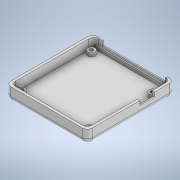
# Autodesk Inventor part: Enclosure Box
Saved by Autodesk Inventor 2021 (Build 250183000, 183)
## iProperties
Created: 2021-06-04
Part Number: Enclosure Box
Material: Generic
Document SubType Name: Modeling
Designer: Anton
Density: 1 g/cm^3
Appearance: Default
Author: Anton
Autodesk Inventor part; units mm, degrees
ref_plane "YZ Plane" through (0, 0, 0) normal (1, 0, 0) x (0, 1, 0)
ref_plane "XZ Plane" through (0, 0, 0) normal (0, 1, 0) x (-1, 0, 0)
ref_plane "XY Plane" through (0, 0, 0) normal (0, 0, 1) x (1, 0, 0)
sketch "Sketch2" plane through (0, 0, 0) normal (0, 1, 0) x (-1, 0, 0)
  line L0 (0, 0) -> (62, 0)
  line L1 (62, 0) -> (62, -66)
  line L2 (62, -66) -> (0, -66)
  line L3 (0, -66) -> (0, 0)
  circle A0 centre (58.15, -9.3) radius 1.5
  circle A1 centre (57.35, -60.86) radius 1.5
  circle A2 centre (3, -4.5) radius 1.5
  circle A3 centre (3, -61.9) radius 1.5
  circle A4 centre (3, -4.5) radius 3
  circle A5 centre (58.15, -9.3) radius 3
  circle A6 centre (57.35, -60.86) radius 3
  circle A7 centre (3, -61.9) radius 3
  line L4 (63, 20) -> (-1, 20)
  line L5 (-1, 20) -> (-1, -86)
  line L6 (-1, -86) -> (63, -86)
  line L7 (63, -86) -> (63, 20)
  dimension "d14" = 66
  dimension "d15" = 62
  dimension "d16" = 3
  dimension "d17" = 3
  dimension "d18" = 3
  dimension "d19" = 3
  dimension "d20" = 3
  dimension "d21" = 4.5
  dimension "d22" = 6
  dimension "d23" = 3
  dimension "d24" = 57.4
  dimension "d25" = 54.35
  dimension "d26" = 0.8
  dimension "d27" = 51.56
  dimension "d28" = 4.8
  dimension "d29" = 6
  dimension "d30" = 6
  dimension "d31" = 6
  dimension "d32" = 20
  dimension "d33" = 20
  dimension "d34" = 1
  dimension "d35" = 1
  constraints: 16 end point, 8 centre point, 4 coincident, 4 parallel, 2 horizontal, 2 perpendicular
  measures "d14" distance between parallel lines of L2 L0
  measures "d15" distance between parallel lines of L3 L1
  measures "d16" diameter of A0
  measures "d17" diameter of A1
  measures "d18" diameter of A3
  measures "d19" diameter of A2
  measures "d20" distance from line of L3 A2.centre
  measures "d21" distance from line of A2.centre L0
  measures "d22" diameter of A4
  measures "d23" distance from line of L3 A3.centre
  measures "d24" distance of A2.centre A3.centre
  measures "d25" horizontal distance of A1.centre A3.centre
  measures "d26" horizontal distance of A1.centre A0.centre
  measures "d27" vertical distance of A1.centre A0.centre
  measures "d28" vertical distance of A2.centre A0.centre
  measures "d29" diameter of A5
  measures "d30" diameter of A6
  measures "d31" diameter of A7
  measures "d32" distance between parallel lines of L4 L0
  measures "d33" distance between parallel lines of L2 L6
  measures "d34" distance between parallel lines of L7 L1
  measures "d35" distance between parallel lines of L3 L5
extrude "Extrusion1" add sketch "Sketch2" along normal blind 2 contours A4 | A7 | L0 L1 L2 L3 | A0 | A1 | A2 | A3 | A5 | A6
sketch "Sketch4" plane through (0, 2, 0) normal (0, 1, 0) x (1, 0, 0)
  line L0 (-62, 66) -> (0, 66)
  line L1 (0, 66) -> (0, 0)
  line L2 (0, 0) -> (-62, 0)
  line L3 (-62, 0) -> (-62, 66)
  circle A0 centre (-3.85, 56.7) radius 1.5
  circle A1 centre (-4.65, 5.14) radius 1.5
  circle A2 centre (-59, 61.5) radius 1.5
  circle A3 centre (-59, 4.1) radius 1.5
  circle A4 centre (-59, 61.5) radius 3
  circle A5 centre (-3.85, 56.7) radius 3
  circle A6 centre (-4.65, 5.14) radius 3
  circle A7 centre (-59, 4.1) radius 3
  point P0 (0, 0)
  dimension "d38" = 66
  dimension "d40" = 3
  dimension "d41" = 3
  dimension "d42" = 3
  dimension "d43" = 3
  dimension "d44" = 3
  dimension "d45" = 4.5
  dimension "d46" = 6
  dimension "d47" = 3
  dimension "d48" = 57.4
  dimension "d50" = 0.8
  dimension "d51" = 51.56
  dimension "d52" = 4.8
  dimension "d53" = 6
  dimension "d54" = 6
  dimension "d55" = 6
  constraints: 8 centre point, 8 end point, 4 coincident, 2 parallel, 1 horizontal, 1 perpendicular
  measures "d38" distance between parallel lines of L2 L0
  measures "d40" diameter of A0
  measures "d41" diameter of A1
  measures "d42" diameter of A3
  measures "d43" diameter of A2
  measures "d44" distance from line of L3 A2.centre
  measures "d45" distance from line of A2.centre L0
  measures "d46" diameter of A4
  measures "d47" distance from line of L3 A3.centre
  measures "d48" distance of A2.centre A3.centre
  measures "d50" horizontal distance of A1.centre A0.centre
  measures "d51" vertical distance of A1.centre A0.centre
  measures "d52" vertical distance of A2.centre A0.centre
  measures "d53" diameter of A5
  measures "d54" diameter of A6
  measures "d55" diameter of A7
extrude "Extrusion2" add sketch "Sketch4" along normal blind 3 contours A4 | A7 | A0 | A1 | A2 | A3 | A5 | A6
sketch "Sketch69" plane through (-59, 5, -4.1) normal (0, 1, 0) x (1, 0, 0)
  circle A0 centre (54.35, 1.04) radius 3 projected
  circle A1 centre (54.35, 1.04) radius 1.25
  circle A2 centre (55.15, 52.6) radius 3 projected
  circle A3 centre (55.15, 52.6) radius 1.25
  circle A4 centre (0, 57.4) radius 3 projected
  circle A5 centre (0, 57.4) radius 1.25
  circle A6 centre (0, 0) radius 3 projected
  circle A7 centre (0, 0) radius 1.25
  point P0 (59, -4.1)
  point P1 (-3, 57.4)
  point P2 (-3, 0)
  dimension "d432" = 2.5
  dimension "d433" = 2.5
  dimension "d434" = 2.5
  dimension "d435" = 2.5
  constraints: 4 centre point, 4 coincident, 2 horizontal alignment
  measures "d432" diameter of A7
  measures "d433" diameter of A5
  measures "d434" diameter of A3
  measures "d435" diameter of A1
extrude "Extrusion56" add sketch "Sketch69" along normal blind 3 contours A1 | A3 | A5 | A7
sketch "Sketch72" plane through (0, 2, 0) normal (0, 1, 0) x (1, 0, 0)
  line L0 (-62, 66) -> (-62, 0) projected
  line L1 (-62, 66) -> (-65, 66)
  line L2 (-65, 66) -> (-65, 0)
  line L3 (-65, 0) -> (-62, 0)
  line L4 (-62, 0) -> (-62, 66)
  circle A0 centre (-59, 61.5) radius 1.25 projected
  line L5 (0, 66) -> (-62, 66) projected
  line L6 (-62, 0) -> (0, 0) projected
  line L7 (0, 0) -> (2.15, 0)
  line L8 (2.15, 0) -> (2.15, 66)
  line L9 (2.15, 66) -> (0, 66)
  line L10 (0, 66) -> (0, 0)
  circle A1 centre (-3.85, 56.7) radius 1.25 projected
  line L11 (-65, 66) -> (2.15, 66)
  line L12 (2.15, 66) -> (2.15, 68.5)
  line L13 (2.15, 68.5) -> (-65, 68.5)
  line L14 (-65, 68.5) -> (-65, 66)
  line L15 (-65, 0) -> (2.15, 0)
  line L16 (2.15, 0) -> (2.15, -3)
  line L17 (2.15, -3) -> (-65, -3)
  line L18 (-65, -3) -> (-65, 0)
  circle A2 centre (-59, 4.1) radius 1.25 projected
  dimension "d446" = 6
  dimension "d447" = 0
  dimension "d448" = 6
  dimension "d449" = 7
  dimension "d450" = 7.1
  dimension "d464" = 0
  dimension "d465" = 0
  constraints: 32 end point, 8 parallel, 4 horizontal, 4 perpendicular, 1 point on line
  measures "d446" distance from line of A0.centre L2
  measures "d447" distance between parallel lines of L5 L1
  measures "d448" distance from line of L8 A1.centre
  measures "d449" distance from line of A0.centre L13
  measures "d450" distance from line of L17 A2.centre
  measures "d464" distance between parallel lines of L8 L12
  measures "d465" distance between parallel lines of L8 L16
extrude "Extrusion58" add sketch "Sketch72" against normal blind 2 contours L0 L3 L2 L1 | L1 L14 L13 L12 L9 L5 | L6 L7 L16 L17 L18 L3 | L9 L8 L7 L10
sketch "Sketch73" plane through (0, 2, 0) normal (0, 1, 0) x (1, 0, 0)
  line L0 (2.15, -3) -> (-65, -3) projected
  line L1 (-65, 68.5) -> (2.15, 68.5) projected
  line L2 (-65, -3) -> (2.15, -3)
  line L3 (2.15, -3) -> (2.15, 68.5)
  line L4 (2.15, 68.5) -> (-65, 68.5)
  line L5 (-65, 68.5) -> (-65, -3)
  line L6 (-63, -1) -> (0.15, -1)
  line L7 (0.15, -1) -> (0.15, 66.5)
  line L8 (0.15, 66.5) -> (-63, 66.5)
  line L9 (-63, 66.5) -> (-63, -1)
  point P0 (0, 0)
  point P1 (2.15, -3)
  dimension "d453" = 2
  constraints: 16 end point, 4 parallel, 2 perpendicular, 1 horizontal, 3 other
  measures "d453" distance between parallel lines of L5 L9
extrude "Extrusion59" add sketch "Sketch73" along normal blind 6
sketch "Sketch74" plane through (0, 8, 0) normal (0, 1, 0) x (1, 0, 0)
  line L0 (6.1553, 52.4) -> (-1.961, 52.4)
  line L1 (-1.961, 52.4) -> (-1.961, 40.4)
  line L2 (-1.961, 40.4) -> (6.1553, 40.4)
  line L3 (6.1553, 40.4) -> (6.1553, 52.4)
  line L4 (-3.5, 77.4858) -> (-56, 77.4858)
  line L5 (-56, 77.4858) -> (-56, 63.7045)
  line L6 (-56, 63.7045) -> (-3.5, 63.7045)
  line L7 (-3.5, 63.7045) -> (-3.5, 77.4858)
  circle A0 centre (-59, 61.5) radius 1.25 projected
  line L8 (0.15, -1) -> (0.15, 66.5) projected
  line L9 (-63, 67.5) -> (0.15, 67.5)
  line L10 (0.15, 67.5) -> (0.15, 64.6943)
  line L11 (0.15, 64.6943) -> (-63, 64.6943)
  line L12 (-63, 64.6943) -> (-63, 67.5)
  line L13 (-63, 66.5) -> (0.15, 66.5) projected
  circle A1 centre (-3.85, 56.7) radius 1.25 projected
  point P0 (0, 0)
  point P1 (-56, 64.6943)
  point P2 (-3.5, 64.6943)
  point P3 (-56, 66.5)
  point P4 (-56, 67.5)
  point P5 (-3.5, 66.5)
  point P6 (0.15, 66.5)
  point P7 (-3.5, 67.5)
  dimension "d457" = 52.5
  dimension "d458" = 1
  dimension "d459" = 4.3
  dimension "d460" = 12
  dimension "d463" = 3
  constraints: 24 end point, 6 parallel, 3 horizontal, 3 perpendicular, 1 point on line
  measures "d457" distance between parallel lines of L7 L5
  measures "d458" distance between parallel lines of L13 L9
  measures "d459" distance from line of L0 A1.centre
  measures "d460" distance between parallel lines of L0 L2
  measures "d463" distance from line of L5 A0.centre
extrude "Extrusion60" cut sketch "Sketch74" against normal blind 3 contours L3 L2 L8 L0 | L8 L2 L1 L0 | L7 L9 L5 L4 | L9 L10 L13 L7 | L7 L13 L5 L9 | L5 L13 L12 L9 | L7 L11 L5 L13
sketch "Sketch75" plane through (0, 5, 0) normal (0, 1, 0) x (1, 0, 0)
  line L0 (-56, 68.5) -> (-3.5, 68.5) projected
  line L1 (-56, 68.5) -> (-3.5, 68.5)
  line L2 (-3.5, 68.5) -> (-3.5, 67.5)
  line L3 (-3.5, 67.5) -> (-56, 67.5)
  line L4 (-56, 67.5) -> (-56, 68.5)
  point P0 (0, 0)
  point P1 (-3.5, 68.5)
  constraints: 8 end point, 2 parallel, 1 horizontal, 1 perpendicular
extrude "Extrusion61" add sketch "Sketch75" along normal blind 1.5
sketch "Sketch77" plane through (0, 5, 0) normal (0, 1, 0) x (1, 0, 0)
  line L0 (2.15, 52.4) -> (2.15, 68.5) projected
  line L1 (2.15, 40.4) -> (0.15, 40.4) projected
  line L2 (2.15, 52.4) -> (1.15, 52.4)
  line L3 (1.15, 52.4) -> (1.15, 40.4)
  line L4 (1.15, 40.4) -> (2.15, 40.4)
  line L5 (2.15, 40.4) -> (2.15, 52.4)
  point P0 (0, 0)
  dimension "d469" = 1
  constraints: 8 end point, 2 parallel, 1 horizontal, 1 midpoint, 1 perpendicular
  measures "d469" distance between parallel lines of L5 L3
extrude "Extrusion62" add sketch "Sketch77" along normal blind 1.5
sketch "Sketch78" plane through (0, 8, 0) normal (0, 1, 0) x (1, 0, 0)
  line L0 (2.15, 40.4) -> (0.15, 40.4) projected
  line L1 (0.15, 40.4) -> (0.15, -1) projected
  line L2 (0.15, -1) -> (-63, -1) projected
  line L3 (-63, -1) -> (-63, 67.5) projected
  line L4 (-63, 67.5) -> (-56, 67.5) projected
  line L5 (-56, 67.5) -> (-56, 68.5) projected
  line L6 (-56, 68.5) -> (-65, 68.5) projected
  line L7 (-65, 68.5) -> (-65, -3) projected
  line L8 (-65, -3) -> (2.15, -3) projected
  line L9 (2.15, -3) -> (2.15, 40.4) projected
  line L10 (0.15, 52.4) -> (2.15, 52.4) projected
  line L11 (2.15, 52.4) -> (2.15, 68.5) projected
  line L12 (2.15, 68.5) -> (-3.5, 68.5) projected
  line L13 (-3.5, 68.5) -> (-3.5, 67.5) projected
  line L14 (-3.5, 67.5) -> (0.15, 67.5) projected
  line L15 (0.15, 67.5) -> (0.15, 52.4) projected
  point P0 (0, 0)
extrude "Extrusion63" add sketch "Sketch78" along normal blind 2
sketch "Sketch80" plane through (0, 10, 0) normal (0, 1, 0) x (1, 0, 0)
  line L0 (2.15, -3) -> (-65, -3) projected
  line L1 (-1.85, -3) -> (-61, -3)
  line L2 (-65, 1) -> (-65, 64.5)
  line L3 (-61, 68.5) -> (-1.85, 68.5)
  line L4 (2.15, 64.5) -> (2.15, 1)
  line L5 (-68.7627, 72.319) -> (6.3795, 72.319)
  line L6 (6.3795, 72.319) -> (6.3795, -5.0493)
  line L7 (6.3795, -5.0493) -> (-68.7627, -5.0493)
  line L8 (-68.7627, -5.0493) -> (-68.7627, 72.319)
  arc A0 (-61, 68.5) -> (-65, 64.5) centre (-61, 64.5) ccw
  arc A1 (2.15, 64.5) -> (-1.85, 68.5) centre (-1.85, 64.5) ccw
  arc A2 (-1.85, -3) -> (2.15, 1) centre (-1.85, 1) ccw
  arc A3 (-65, 1) -> (-61, -3) centre (-61, 1) ccw
  point P0 (0, 0)
  point P1 (-65, 68.5)
  dimension "d475" = 4
  constraints: 16 end point, 8 point on circle, 8 tangent, 4 centre point, 4 parallel, 4 point on line, 3 equal radius, 2 horizontal, 2 perpendicular
  measures "d475" radius of A0
extrude "Extrusion64" cut sketch "Sketch80" against normal blind 10
sketch "Sketch81" plane through (0, 10, 0) normal (0, 1, 0) x (1, 0, 0)
  line L0 (0.15, 40.4) -> (0.15, -1) projected
  line L1 (-63, 66.5) -> (-63, 67.5) projected
  line L2 (-3.85, -1) -> (-59, -1)
  line L3 (-63, 3) -> (-63, 63.5)
  line L4 (-59, 67.5) -> (-3.85, 67.5)
  line L5 (0.15, 63.5) -> (0.15, 3)
  arc A0 (-59, 67.5) -> (-63, 63.5) centre (-59, 63.5) ccw
  arc A1 (0.15, 63.5) -> (-3.85, 67.5) centre (-3.85, 63.5) ccw
  arc A2 (-3.85, -1) -> (0.15, 3) centre (-3.85, 3) ccw
  arc A3 (-63, 3) -> (-59, -1) centre (-59, 3) ccw
  line L6 (0.15, -1) -> (-63, -1) projected
  line L7 (-63, 67.5) -> (0.15, 67.5)
  line L8 (0.15, 67.5) -> (0.15, -1)
  line L9 (0.15, -1) -> (-63, -1)
  line L10 (-63, -1) -> (-63, 67.5)
  point P0 (0, 0)
  dimension "d478" = 4
  constraints: 16 end point, 8 point on circle, 8 tangent, 4 centre point, 4 parallel, 4 point on line, 3 equal radius, 2 horizontal, 2 perpendicular
  measures "d478" radius of A0
extrude "Extrusion65" add sketch "Sketch81" against normal up to surface (8 mm away) contours L0 L6 A2 | A1 L7 L8 | L6 L10 A3 | A0 L10 L1 L7
sketch "Sketch82" plane through (0, 0, 0) normal (0, -1, 0) x (1, 0, 0)
  arc A0 (-61, 3) -> (-65, -1) centre (-61, -1) ccw projected
  line L0 (-65, -1) -> (-65, -64.5) projected
  arc A1 (-65, -64.5) -> (-61, -68.5) centre (-61, -64.5) ccw projected
  line L1 (-61, -68.5) -> (-1.85, -68.5) projected
  arc A2 (-1.85, -68.5) -> (2.15, -64.5) centre (-1.85, -64.5) ccw projected
  line L2 (2.15, -64.5) -> (2.15, -1) projected
  arc A3 (2.15, -1) -> (-1.85, 3) centre (-1.85, -1) ccw projected
  line L3 (-1.85, 3) -> (-61, 3) projected
  point P0 (0, 0)
extrude "Extrusion66" add sketch "Sketch82" along normal blind 1
sketch "Sketch83" plane through (-59, 5, -4.1) normal (0, 1, 0) x (1, 0, 0)
  circle A0 centre (54.35, 1.04) radius 1.25 projected
  circle A1 centre (54.35, 1.04) radius 1.5
  circle A2 centre (55.15, 52.6) radius 1.25 projected
  circle A3 centre (55.15, 52.6) radius 1.5
  circle A4 centre (0, 57.4) radius 1.25 projected
  circle A5 centre (0, 57.4) radius 1.5
  circle A6 centre (0, 0) radius 1.25 projected
  circle A7 centre (0, 0) radius 1.5
  point P0 (59, -4.1)
  dimension "d484" = 3
  dimension "d486" = 3
  dimension "d487" = 3
  dimension "d488" = 3
  constraints: 4 centre point, 4 coincident
  measures "d484" diameter of A7
  measures "d486" diameter of A5
  measures "d487" diameter of A3
  measures "d488" diameter of A1
extrude "Extrusion67" cut sketch "Sketch83" along normal mid plane 1011 contours A0 | A1 | A2 | A3 | A4 | A5 | A6 | A7
fillet "Fillet13" radius 4 8 edges at (0.9784, -1, -67.3284) (2.15, -1, -32.75) (0.9784, -1, 1.8284) (-31.425, -1, 3) (-63.8284, -1, 1.8284) (-65, -1, -32.75) (-63.8284, -1, -67.3284) (-31.425, -1, -68.5)
sketch "Sketch84" plane through (0, -1, 0) normal (0, -1, 0) x (1, 0, 0)
  circle A0 centre (-4.65, -5.14) radius 3 projected
  circle A1 centre (-4.65, -5.14) radius 3
  circle A2 centre (-3.85, -56.7) radius 1.5 projected
  circle A3 centre (-3.85, -56.7) radius 3
  circle A4 centre (-59, -61.5) radius 1.5 projected
  circle A5 centre (-59, -61.5) radius 3
  circle A6 centre (-59, -4.1) radius 1.5 projected
  circle A7 centre (-59, -4.1) radius 3
  point P0 (0, 0)
  dimension "d492" = 6
  dimension "d493" = 6
  dimension "d494" = 6
  dimension "d495" = 6
  constraints: 4 centre point, 4 coincident
  measures "d492" diameter of A7
  measures "d493" diameter of A5
  measures "d494" diameter of A3
  measures "d495" diameter of A1
extrude "Extrusion68" cut sketch "Sketch84" against normal blind 2.5 contours A0 | A2 | A3 | A4 | A5 | A7
body "Solid1"
